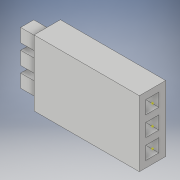
# Autodesk Inventor part: konektorservomotora
Saved by Autodesk Inventor 2019 (Build 230136000, 136)
## iProperties
Created: 2018-12-19
Part Number: konektorservomotora
Material: Generic
Document SubType Name: Modeling
Designer: nikol
Density: 1 g/cm^3
Appearance: Default
Author: nikol
Autodesk Inventor part; units mm, degrees
ref_plane "YZ Plane" through (0, 0, 0) normal (1, 0, 0) x (0, 1, 0)
ref_plane "XZ Plane" through (0, 0, 0) normal (0, 1, 0) x (-1, 0, 0)
ref_plane "XY Plane" through (0, 0, 0) normal (0, 0, 1) x (1, 0, 0)
sketch "Sketch1" plane through (0, 0, 0) normal (1, 0, 0) x (0, 1, 0)
  line L0 (3.5, 1) -> (-1.5, 1)
  line L1 (-1.5, 1) -> (-1.5, -1)
  line L2 (-1.5, -1) -> (3.5, -1)
  line L3 (3.5, -1) -> (3.5, 1)
  point P0 (0, 0)
  dimension "d0" = 2
  dimension "d1" = 5
  dimension "d2" = 3.5
  dimension "d3" = 1
  constraints: 8 end point, 2 parallel, 1 horizontal, 1 perpendicular
  measures "d0" distance of L2.end L0.start
  measures "d1" distance of L1.end L2.end
  measures "d2" distance from line of L3 point (0, 0)
  measures "d3" distance from line of L0 point (0, 0)
extrude "Extrusion1" add sketch "Sketch1" along normal blind 8
sketch "Sketch2" plane through (8, 0, 0) normal (1, 0, 0) x (0, 0, -1)
  line L0 (-0.5192, 3) -> (0.4808, 3)
  line L1 (0.4808, 3) -> (0.4808, 2)
  line L2 (0.4808, 2) -> (-0.5192, 2)
  line L3 (-0.5192, 2) -> (-0.5192, 3)
  line L4 (-0.5192, 1.5) -> (0.4808, 1.5)
  line L5 (0.4808, 1.5) -> (0.4808, 0.5)
  line L6 (0.4808, 0.5) -> (-0.5192, 0.5)
  line L7 (-0.5192, 0.5) -> (-0.5192, 1.5)
  line L8 (-0.5192, 0) -> (0.4808, 0)
  line L9 (0.4808, 0) -> (0.4808, -1)
  line L10 (0.4808, -1) -> (-0.5192, -1)
  line L11 (-0.5192, -1) -> (-0.5192, 0)
  line L12 (1, 3.5) -> (-1, 3.5) projected
  point P0 (0, 0)
  dimension "d6" = 1
  dimension "d7" = 1
  dimension "d8" = 1
  dimension "d9" = 1
  dimension "d10" = 1
  dimension "d11" = 0.5
  dimension "d12" = 0.5
  dimension "d13" = 0.5
  constraints: 24 end point, 6 parallel, 4 point on line, 3 horizontal, 3 perpendicular
  measures "d6" distance of L0.start L0.end
  measures "d7" distance of L0.end L1.end
  measures "d8" distance of L4.start L4.end
  measures "d9" distance of L4.end L5.end
  measures "d10" distance of L8.end L9.end
  measures "d11" distance between parallel lines of L12 L0
  measures "d12" distance between parallel lines of L4 L2
  measures "d13" distance between parallel lines of L8 L6
extrude "Extrusion2" cut sketch "Sketch2" against normal blind 5
sketch "Sketch3" plane through (0, 0, 0) normal (-1, 0, 0) x (0, 0, 1)
  line L0 (-0.4808, 0) -> (-0.4808, -1) projected
  line L1 (0.5192, -1) -> (0.5192, 0) projected
  line L2 (-0.4808, -1) -> (0.5192, -1)
  line L3 (0.5192, -1) -> (0.5192, 0)
  line L4 (0.5192, 0) -> (-0.4808, 0)
  line L5 (-0.4808, 0) -> (-0.4808, -1)
  line L6 (-0.4808, 1.5) -> (-0.4808, 0.5) projected
  line L7 (0.5192, 1.5) -> (-0.4808, 1.5) projected
  line L8 (-0.4808, 0.5) -> (0.5192, 0.5)
  line L9 (0.5192, 0.5) -> (0.5192, 1.5)
  line L10 (0.5192, 1.5) -> (-0.4808, 1.5)
  line L11 (-0.4808, 1.5) -> (-0.4808, 0.5)
  line L12 (0.5192, 2) -> (0.5192, 3) projected
  line L13 (-0.4808, 1.9917) -> (0.5192, 1.9917)
  line L14 (0.5192, 1.9917) -> (0.5192, 3)
  line L15 (0.5192, 3) -> (-0.4808, 3)
  line L16 (-0.4808, 3) -> (-0.4808, 1.9917)
  point P0 (0, 0)
  constraints: 24 end point, 6 parallel, 3 horizontal, 3 perpendicular, 1 point on line
extrude "Extrusion3" add sketch "Sketch3" along normal blind 1.5
body "Solid1"
